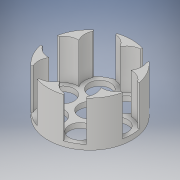
# Autodesk Inventor part: hand_joy_cover
Saved by Autodesk Inventor 2019 (Build 230136000, 136)
## iProperties
Created: 2018-11-04
Part Number: hand_joy_cover
Material: 일반
Document SubType Name: Modeling
Designer: otm09
Density: 1 g/cm^3
Appearance: 기본값
Author: otm09
Autodesk Inventor part; units mm, degrees
ref_plane "YZ Plane" through (0, 0, 0) normal (1, 0, 0) x (0, 1, 0)
ref_plane "XZ Plane" through (0, 0, 0) normal (0, 1, 0) x (-1, 0, 0)
ref_plane "XY Plane" through (0, 0, 0) normal (0, 0, 1) x (1, 0, 0)
sketch "스케치1" plane through (0, 0, 0) normal (0, 1, 0) x (-1, 0, 0)
  circle A0 centre (0, 0) radius 25
  circle A1 centre (16, 0) radius 6.5
  circle A2 centre (8, 13.8564) radius 6.5
  circle A3 centre (-8, 13.8564) radius 6.5
  circle A4 centre (-16, 0) radius 6.5
  circle A5 centre (-8, -13.8564) radius 6.5
  circle A6 centre (8, -13.8564) radius 6.5
  circle A7 centre (0, 0) radius 6.5
  dimension "d0" = 50
  dimension "d1" = 13
  dimension "d2" = 16
  dimension "d5" = 360
  dimension "d7" = 13
  constraints: 8 centre point, 2 coincident, 13 other
  measures "d0" diameter of A0
  measures "d1" diameter of A1
  measures "d2" distance of A0.centre A1.centre
  measures "d7" diameter of A7
extrude "돌출1" add sketch "스케치1" along normal blind 3
sketch "스케치2" plane through (0, 3, 0) normal (0, 1, 0) x (1, 0, 0)
  circle A0 centre (-16, 0) radius 6.5 projected
  circle A1 centre (-8, 13.8564) radius 6.5 projected
  circle A2 centre (8, 13.8564) radius 6.5 projected
  circle A3 centre (8, -13.8564) radius 6.5 projected
  circle A4 centre (-8, -13.8564) radius 6.5 projected
  circle A5 centre (0, 0) radius 25
  arc A6 (-15.5707, 8.9898) -> (-15.5707, -8.9898) centre (-16, 0) ccw
  arc A7 (0, 17.9795) -> (-15.5707, 8.9898) centre (-8, 13.8564) ccw
  arc A8 (15.5707, 8.9898) -> (0, 17.9795) centre (8, 13.8564) ccw
  arc A9 (15.5707, -8.9898) -> (15.5707, 8.9898) centre (16, 0) ccw
  arc A10 (0, -17.9795) -> (15.5707, -8.9898) centre (8, -13.8564) ccw
  arc A11 (-15.5707, -8.9898) -> (0, -17.9795) centre (-8, -13.8564) ccw
  line L0 (25, -5) -> (-25, -5)
  line L1 (-25, -5) -> (-25, 5)
  line L2 (-25, 5) -> (25, 5)
  line L3 (25, 5) -> (25, -5)
  line L4 (25, -5) -> (-25, 5) construction
  line L5 (-25, -5) -> (25, 5) construction
  line L6 (-8.1699, -24.1506) -> (-16.8301, -19.1506)
  line L7 (-16.8301, -19.1506) -> (8.1699, 24.1506)
  line L8 (16.8301, 19.1506) -> (-8.1699, -24.1506)
  line L9 (8.1699, 24.1506) -> (16.8301, 19.1506)
  line L10 (16.8301, -19.1506) -> (8.1699, -24.1506)
  line L11 (8.1699, -24.1506) -> (-16.8301, 19.1506)
  line L12 (-8.1699, 24.1506) -> (16.8301, -19.1506)
  line L13 (-16.8301, 19.1506) -> (-8.1699, 24.1506)
  line L14 (25, 5) -> (25, -5)
  line L15 (25, -5) -> (-25, -5)
  line L16 (-25, 5) -> (25, 5)
  line L17 (-25, -5) -> (-25, 5)
  line L18 (8.1699, 24.1506) -> (16.8301, 19.1506)
  line L19 (16.8301, 19.1506) -> (-8.1699, -24.1506)
  line L20 (-16.8301, -19.1506) -> (8.1699, 24.1506)
  line L21 (-8.1699, -24.1506) -> (-16.8301, -19.1506)
  line L22 (-16.8301, 19.1506) -> (-8.1699, 24.1506)
  line L23 (-8.1699, 24.1506) -> (16.8301, -19.1506)
  line L24 (8.1699, -24.1506) -> (-16.8301, 19.1506)
  line L25 (16.8301, -19.1506) -> (8.1699, -24.1506)
  point P0 (16, 0)
  dimension "d17" = 50
  dimension "d18" = 10
  dimension "d21" = 360
  constraints: 52 end point, 12 point on circle, 7 centre point, 2 midpoint, 2 parallel, 1 perpendicular, 49 other
  measures "d17" distance of L0.start L0.end
  measures "d18" distance of L0.end L1.end
extrude "돌출2" add sketch "스케치2" along normal blind 24 contours L2 A5 L11 A7 A6 | A6 A5 L2 | L0 A5 A6 | A6 A11 L7 A5 L0 | L11 A5 A7 | A11 A5 L7 | A5 L12 A7 | L2 A5 A9 | A9 A8 L8 A5 L2 | L12 A5 L7 A8 A7 | A11 L8 A5 | L0 A5 L12 A10 A9 | A9 A5 L0 | A11 A10 L11 A5 L8 | L7 A5 A8 | A10 A5 L11 | A8 A5 L8 | L12 A5 A10
extrude "돌출3" cut sketch "스케치2" along normal blind 27 contours A0 L0 L2 | A0 L2 L11 L7 L0 | A0 L0 A6 L2 | L11 A1 L12 L7 L2 | L2 L7 L11 | L7 L11 L0 | L0 L11 L8 A4 L7 | A6 A5 L2 | L7 L12 L2 | L2 L12 L8 L0 L11 L7 | L11 A1 L12 | L0 A5 A6 | L0 L8 L11 | A4 L8 L7 | L1 L2 A5 | A5 L0 L1 | L12 L7 A2 L8 L2 | L2 L8 L12 | L11 A7 L12 A1 | L8 L12 L0 | L0 L12 A3 L11 L8 | A4 L8 A11 L7 | L11 A5 A7 | L11 L13 A5 | L2 A9 L0 L12 L8 | L7 A2 L8 | A11 A5 L7 | A5 L6 L7 | A3 L12 L11 | L13 L12 A5 | A5 L12 A7 | L2 A5 A9 | L7 A8 L8 A2 | A11 L8 A5 | A5 L8 L6 | A9 A5 L0 | A3 L12 A10 L11 | L3 L0 A5 | A5 L2 L3 | L7 A5 A8 | A10 A5 L11 | L7 L9 A5 | A8 A5 L8 | A5 L9 L8 | A5 L10 L11 | L12 A5 A10 | L12 L10 A5
